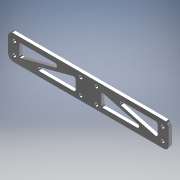
# Autodesk Inventor part: Back Plate Spinning thing
Saved by Autodesk Inventor 2019.4 (Build 234330000, 330)
## iProperties
Created: 2020-01-23
Part Number: Back Plate Spinning thing
Material: Aluminum 6061
Document SubType Name: Modeling
Designer: Mark
Mass: 127.034 g
Surface Area: 223.11 cm^2
Volume: 47.0497 cm^3
Density: 2.7 g/cm^3
Appearance: Aluminum - Flat
Author: Mark
Autodesk Inventor part; units mm, degrees
ref_plane "YZ Plane" through (0, 0, 0) normal (1, 0, 0) x (0, 1, 0)
ref_plane "XZ Plane" through (0, 0, 0) normal (0, 1, 0) x (-1, 0, 0)
ref_plane "XY Plane" through (0, 0, 0) normal (0, 0, 1) x (1, 0, 0)
sketch "Sketch1" plane through (0, 0, 0) normal (0, 0, 1) x (1, 0, 0)
  line L0 (-139.5, -20) -> (139.5, -20)
  line L1 (139.5, -20) -> (139.5, 20)
  line L2 (139.5, 20) -> (-139.5, 20)
  line L3 (-139.5, 20) -> (-139.5, -20)
  line L4 (-139.5, -20) -> (139.5, 20) construction
  line L5 (139.5, -20) -> (-139.5, 20) construction
  line L6 (12.7, -12.7) -> (-12.7, -12.7) construction
  line L7 (-12.7, -12.7) -> (-12.7, 12.7) construction
  line L8 (-12.7, 12.7) -> (12.7, 12.7) construction
  line L9 (12.7, 12.7) -> (12.7, -12.7) construction
  line L10 (12.7, -12.7) -> (-12.7, 12.7) construction
  line L11 (-12.7, -12.7) -> (12.7, 12.7) construction
  circle A0 centre (-12.7, 12.7) radius 2.75
  circle A1 centre (12.7, 12.7) radius 2.75
  circle A2 centre (12.7, -12.7) radius 2.75
  circle A3 centre (-12.7, -12.7) radius 2.75
  circle A4 centre (-129.5, 10) radius 2.75
  circle A5 centre (-129.5, -10) radius 2.75
  circle A6 centre (129.5, 10) radius 2.75
  circle A7 centre (129.5, -10) radius 2.75
  point P0 (0, 0)
  dimension "d0" = 279
  dimension "d1" = 40
  dimension "d2" = 25.4
  dimension "d3" = 25.4
  dimension "d4" = 5.5
  dimension "d5" = 5.5
  dimension "d6" = 5.5
  dimension "d7" = 5.5
  dimension "d8" = 5.5
  dimension "d9" = 5.5
  dimension "d10" = 5.5
  dimension "d11" = 5.5
  dimension "d12" = 10
  dimension "d13" = 10
  dimension "d14" = 10
  dimension "d15" = 10
  dimension "d16" = 10
  dimension "d17" = 10
  dimension "d18" = 10
  dimension "d19" = 10
  constraints: 24 end point, 8 centre point, 4 coincident, 4 midpoint, 4 parallel, 2 horizontal, 2 perpendicular
  measures "d0" distance of L2.end L1.end
  measures "d1" distance of L1.end L0.end
  measures "d2" distance of L7.end L8.end
  measures "d3" distance of L6.end L7.end
  measures "d4" diameter of A0
  measures "d5" diameter of A1
  measures "d6" diameter of A2
  measures "d7" diameter of A3
  measures "d8" diameter of A4
  measures "d9" diameter of A5
  measures "d10" diameter of A6
  measures "d11" diameter of A7
  measures "d12" distance from line of L0 A7.centre
  measures "d13" distance from line of L2 A6.centre
  measures "d14" distance from line of L2 A4.centre
  measures "d15" distance from line of L0 A5.centre
  measures "d16" distance from line of L3 A4.centre
  measures "d17" distance from line of L3 A5.centre
  measures "d18" distance from line of L1 A7.centre
  measures "d19" distance from line of L1 A6.centre
extrude "Extrusion1" add sketch "Sketch1" along normal blind 5
fillet "Fillet1" radius 8 4 edges at (139.5, 20, 2.5) (139.5, -20, 2.5) (-139.5, 20, 2.5) (-139.5, -20, 2.5)
sketch "Sketch2" plane through (0, 0, 5) normal (0, 0, 1) x (1, 0, 0)
  line L0 (-121.5, 12) -> (-31.4935, 12)
  line L1 (-20.7, 12) -> (-20.7, 9.4301) construction
  line L2 (-20.7, -12) -> (-110.7065, -12)
  line L3 (-121.5, -12) -> (-121.5, -9.4301) construction
  line L4 (131.5, 20) -> (-131.5, 20) projected
  line L5 (-131.5, -20) -> (131.5, -20) projected
  circle A0 centre (-129.5, -10) radius 2.75 projected
  circle A1 centre (-12.7, -12.7) radius 2.75 projected
  line L6 (-121.5, -9.4301) -> (-31.4935, 12)
  line L7 (-20.7, 9.4301) -> (-110.7065, -12)
  line L8 (-121.5, -12) -> (-20.7, 12) construction
  line L9 (0, -20) -> (0, 20)
  line L10 (121.5, 12) -> (31.4935, 12)
  line L11 (20.7, 12) -> (20.7, 9.4301) construction
  line L12 (20.7, -12) -> (110.7065, -12)
  line L13 (121.5, -12) -> (121.5, -9.4301) construction
  line L14 (121.5, -9.4301) -> (31.4935, 12)
  line L15 (20.7, 9.4301) -> (110.7065, -12)
  line L16 (-121.5, -9.4301) -> (-121.5, 12)
  line L17 (-110.7065, -12) -> (-121.5, -12) construction
  line L18 (-31.4935, 12) -> (-20.7, 12) construction
  line L19 (-20.7, 9.4301) -> (-20.7, -12)
  line L20 (31.4935, 12) -> (20.7, 12) construction
  line L21 (20.7, 9.4301) -> (20.7, -12)
  line L22 (121.5, -9.4301) -> (121.5, 12)
  line L23 (110.7065, -12) -> (121.5, -12) construction
  point P0 (0, 0)
  dimension "d23" = 8
  dimension "d24" = 8
  dimension "d25" = 8
  dimension "d26" = 8
  dimension "d31" = 5
  dimension "d32" = 2.5
  constraints: 44 end point, 10 parallel, 8 symmetric about line, 4 perpendicular, 2 horizontal, 2 midpoint
  measures "d23" distance between parallel lines of L4 L0
  measures "d24" distance between parallel lines of L5 L2
  measures "d25" distance from line of A0.centre L3
  measures "d26" distance from line of L1 A1.centre
  measures "d31" distance between parallel lines of L7 L6
  measures "d32" distance between parallel lines of L6 L8
extrude "Extrusion2" cut sketch "Sketch2" against normal through all contours L0 L6 L16 | L2 L7 L19 | L22 L14 L10 | L21 L15 L12
fillet "Fillet2" radius 3 12 edges at (-121.5, -9.4301, 2.5) (-121.5, 12, 2.5) (-31.4935, 12, 2.5) (-110.7065, -12, 2.5) (-20.7, -12, 2.5) (-20.7, 9.4301, 2.5) (20.7, 9.4301, 2.5) (20.7, -12, 2.5) (110.7065, -12, 2.5) (121.5, -9.4301, 2.5) (31.4935, 12, 2.5) (121.5, 12, 2.5)
body "Solid1"
